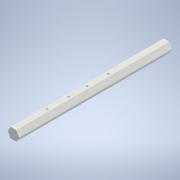
# Autodesk Inventor part: Eje2
Saved by Autodesk Inventor 2022 (Build 260153000, 153)
## iProperties
Created: 2022-02-21
Part Number: Eje2
Material: Generic
Document SubType Name: Modeling
Designer: katha
Density: 1 g/cm^3
Appearance: Default
Author: katha
Autodesk Inventor part; units mm, degrees
ref_plane "YZ Plane" through (0, 0, 0) normal (1, 0, 0) x (0, 1, 0)
ref_plane "XZ Plane" through (0, 0, 0) normal (0, 1, 0) x (-1, 0, 0)
ref_plane "XY Plane" through (0, 0, 0) normal (0, 0, 1) x (1, 0, 0)
sketch "Sketch1" plane through (0, 0, 0) normal (0, 0, 1) x (1, 0, 0)
  line L0 (3, 0) -> (1.5, -2.5981) projected
  line L1 (1.5, -2.5981) -> (-1.5, -2.5981) projected
  line L2 (-1.5, -2.5981) -> (-3, 0) projected
  line L3 (-3, 0) -> (-1.5, 2.5981) projected
  line L4 (-1.5, 2.5981) -> (1.5, 2.5981) projected
  line L5 (1.5, 2.5981) -> (3, 0) projected
  point P0 (0, 0)
extrude "Extrusion1" add sketch "Sketch1" along normal blind 80
sketch "Sketch2" plane through (-1.5, 2.5981, 0) normal (0, 1, 0) x (1, 0, 0)
  circle A0 centre (1.5, -30.5) radius 0.625 projected
  circle A1 centre (1.5, -41.7) radius 0.625 projected
  circle A2 centre (1.5, -51.3) radius 0.625 projected
  circle A3 centre (1.5, -62.5) radius 0.625 projected
  point P0 (1.5, 0)
extrude "Extrusion2" cut sketch "Sketch2" against normal blind 10
body "Solid1"
